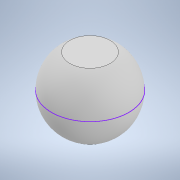
# Autodesk Inventor part: solid mid ball
Saved by Autodesk Inventor 2022 (Build 260153000, 153)
## iProperties
Created: 2022-03-15
Part Number: solid mid ball
Material: Generic
Document SubType Name: Modeling
Designer: mogje
Density: 1 g/cm^3
Appearance: Default
Author: mogje
Autodesk Inventor part; units mm, degrees
ref_plane "YZ Plane" through (0, 0, 0) normal (1, 0, 0) x (0, 1, 0)
ref_plane "XZ Plane" through (0, 0, 0) normal (0, 1, 0) x (-1, 0, 0)
ref_plane "XY Plane" through (0, 0, 0) normal (0, 0, 1) x (1, 0, 0)
sketch "Sketch3" plane through (0, 0, 0) normal (1, 0, 0) x (0, 1, 0)
  line L0 (-27.1198, 0) -> (-27.1198, -16.51)
  line L1 (27.1198, 0) -> (27.1198, -16.51)
  arc A0 (-27.1198, -16.51) -> (27.1198, -16.51) centre (0, 0) ccw
  line L2 (27.1198, 0) -> (-27.1198, 0)
  constraints: 6 end point, 2 point on circle, 2 vertical, 1 centre point, 1 coincident
revolve "Revolution2" add sketch "Sketch3" angle 360 about axis through (0, 27.1198, 0) along (0, -1, 0)
sketch "Sketch4" plane through (0, 0, 0) normal (0, 1, 0) x (-1, 0, 0)
  circle A0 centre (0, 0) radius 31.75
  constraints: 1 centre point, 1 coincident
body "Solid2"
